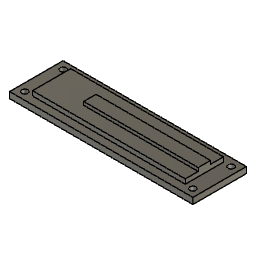
Suporte_encaixe (Autodesk Fusion 360 design; units mm, degrees)
Autodesk Fusion 360 part; units mm, degrees
sketch "Esboço1" plane through (0, 0, 0) normal (0, 0, 1) x (1, 0, 0)
  line L0 (0, 0) -> (120, 0)
  line L1 (120, 0) -> (120, 35)
  line L2 (120, 35) -> (0, 35)
  line L3 (0, 35) -> (0, 0)
  dimension "d1" = 120
  dimension "d2" = 35
  constraint horizontal L0
  constraint vertical L1
  constraint horizontal L2
  constraint vertical L3
  constraint coincident L0.start L3.end
  measures "d1" distance of L0.start L0.end
  measures "d2" distance of L0.start L2.end
extrude "Extrusão1" add sketch "Esboço1" along normal blind 4
sketch "Esboço2" plane through (0, 0, 4) normal (0, 0, 1) x (-1, 0, 0)
  line L0 (0, -35) -> (0, 0)
  line L1 (0, 0) -> (-120, 0)
  line L2 (-120, 0) -> (-120, -35)
  line L3 (-120, -35) -> (0, -35)
  line L4 (-10, -30) -> (-110, -30)
  line L5 (-110, -30) -> (-110, -5)
  line L6 (-110, -5) -> (-10, -5)
  line L7 (-10, -5) -> (-10, -30)
  point P0 (-5, -30)
  point P1 (-5, -5)
  point P2 (-115, -5)
  point P3 (-115, -30)
  constraint horizontal L4
  constraint vertical L5
  constraint horizontal L6
  constraint vertical L7
sketch "Esboço8" plane through (0, 0, 4) normal (0, 0, 1) x (1, 0, 0)
  circle A0 centre (5, 30) radius 2
  circle A1 centre (5, 5) radius 2
  circle A2 centre (115, 30) radius 2
  circle A3 centre (115, 5) radius 2
  dimension "d18" = 4
  dimension "d19" = 4
  dimension "d20" = 4
  dimension "d21" = 4
  measures "d18" diameter of A0
  measures "d19" diameter of A1
  measures "d20" diameter of A2
  measures "d21" diameter of A3
extrude "Extrusão7" cut sketch "Esboço8" against normal blind 20
extrude "Extrusão10" add sketch "Esboço2" along normal blind 3 contours L4 L5 L6 L7
sketch "Esboço10" plane through (0, 0, 7) normal (0, 0, 1) x (-1, 0, 0)
  line L0 (-10, -5) -> (-110, -5)
  line L1 (-110, -5) -> (-110, -30)
  line L2 (-110, -30) -> (-10, -30)
  line L3 (-10, -30) -> (-10, -5)
  line L4 (-110, -30) -> (-110, -21.55)
  line L5 (-110, -5) -> (-110, -13.45)
  line L6 (-110, -21.55) -> (-35.05, -21.55)
  line L7 (-110, -13.45) -> (-35.05, -13.45)
  line L8 (-35.05, -21.55) -> (-35.05, -13.45)
  dimension "d35" = 8.45
  dimension "d36" = 8.45
  dimension "d37" = 74.95
  dimension "d38" = 74.95
  constraint coincident L1.end L2.start
  constraint perpendicular L2 L4
  constraint coincident L0.end L1.start
  constraint perpendicular L0 L5
  constraint perpendicular L4 L6
  constraint perpendicular L5 L7
  measures "d35" distance of L1.end L4.end
  measures "d36" distance of L0.end L5.end
  measures "d37" distance of L4.end L6.end
  measures "d38" distance of L5.end L7.end
extrude "Extrusão11" add sketch "Esboço10" along normal blind 2.2 contours L1 L6 L7 L8
